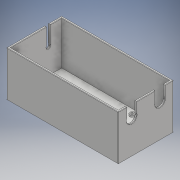
# Autodesk Inventor part: END NODE SIMPLE
Saved by Autodesk Inventor 2017 (Build 210142000, 142)
## iProperties
Created: 2019-07-16
Part Number: END NODE SIMPLE
Material: Generic
Document SubType Name: Modeling
Designer: harneet
Density: 1 g/cm^3
Appearance: Default
Author: harneet
Autodesk Inventor part; units mm, degrees
ref_plane "YZ Plane" through (0, 0, 0) normal (1, 0, 0) x (0, 1, 0)
ref_plane "XZ Plane" through (0, 0, 0) normal (0, 1, 0) x (-1, 0, 0)
ref_plane "XY Plane" through (0, 0, 0) normal (0, 0, 1) x (1, 0, 0)
sketch "Sketch1" plane through (0, 0, 0) normal (0, 0, 1) x (1, 0, 0)
  line L0 (-68.5, 32.5) -> (68.5, 32.5)
  line L1 (68.5, 32.5) -> (68.5, -32.5)
  line L2 (68.5, -32.5) -> (-68.5, -32.5)
  line L3 (-68.5, -32.5) -> (-68.5, 32.5)
  line L4 (71, 35) -> (-71, 35)
  line L5 (-71, 35) -> (-71, -35)
  line L6 (-71, -35) -> (71, -35)
  line L7 (71, -35) -> (71, 35)
  point P0 (0, 0)
  dimension "d0" = 137
  dimension "d1" = 68.5
  dimension "d2" = 65
  dimension "d3" = 32.5
  dimension "d4" = 2.5
  constraints: 16 end point, 4 parallel, 2 perpendicular, 1 horizontal, 3 other
  measures "d0" distance of L0.start L0.end
  measures "d1" distance from line of point (0, 0) L3
  measures "d2" distance of L2.end L0.start
  measures "d3" distance from line of L2 point (0, 0)
  measures "d4" distance between parallel lines of L0 L4
extrude "Extrusion1" add sketch "Sketch1" along normal blind 55
sketch "Sketch2" plane through (0, 0, 0) normal (0, 0, -1) x (-1, 0, 0)
  line L0 (71, 35) -> (-71, 35)
  line L1 (-71, 35) -> (-71, -35)
  line L2 (-71, -35) -> (71, -35)
  line L3 (71, -35) -> (71, 35)
  point P0 (0, 0)
  dimension "d7" = 142
  dimension "d8" = 70
  dimension "d9" = 35
  dimension "d10" = 71
  constraints: 8 end point, 2 parallel, 1 horizontal, 1 perpendicular
  measures "d7" distance of L1.end L2.end
  measures "d8" distance of L0.end L1.end
  measures "d9" distance from line of point (0, 0) L2
  measures "d10" distance from line of point (0, 0) L1
extrude "Extrusion2" add sketch "Sketch2" along normal blind 2.5
sketch "Sketch3" plane through (71, -35, 55) normal (1, 0, 0) x (0, 0, -1)
  circle A0 centre (15, 17) radius 6.375
  circle A1 centre (15, 53) radius 6.375
  line L0 (55, 2.5) -> (55, 67.5) projected
  line L1 (57.5, 0) -> (0, 0) projected
  point P0 (55, 35)
  dimension "d13" = 12.75
  dimension "d14" = 12.75
  dimension "d15" = 40
  dimension "d16" = 40
  dimension "d17" = 36
  dimension "d18" = 17
  constraints: 2 centre point
  measures "d13" diameter of A0
  measures "d14" diameter of A1
  measures "d15" distance from line of L0 A0.centre
  measures "d16" distance from line of A1.centre L0
  measures "d17" distance of A1.centre A0.centre
  measures "d18" distance from line of L1 A0.centre
extrude "Extrusion3" cut sketch "Sketch3" against normal up to surface (2.5 mm away)
sketch "Sketch4" plane through (-68.5, -32.5, 55) normal (1, 0, 0) x (0, 0, -1)
  circle A0 centre (23, 48) radius 2.5
  circle A1 centre (15, 50.5) radius 6.375 projected
  point P0 (55, 32.5)
  point P1 (0, 65)
  dimension "d21" = 5
  dimension "d22" = 17
  dimension "d25" = 8
  constraints: 1 centre point
  measures "d21" diameter of A0
  measures "d22" vertical distance of point (0, 65) A0.centre
  measures "d25" horizontal distance of A0.centre A1.centre
extrude "Extrusion4" cut sketch "Sketch4" against normal blind 2.5 contours A0 A1 | A1 A0 picked at (22.5229, 48.2025) picked at (20.8961, 48.5627)
sketch "Sketch5" plane through (0, 0, 0) normal (0, 0, 1) x (1, 0, 0)
  circle A0 centre (28.5, -7) radius 1.5
  circle A1 centre (28.5, -22.5) radius 1.5
  line L0 (68.5, 32.5) -> (68.5, -32.5) projected
  line L1 (68.5, -32.5) -> (-68.5, -32.5) projected
  point P0 (0, 0)
  dimension "d28" = 3
  dimension "d29" = 3
  dimension "d32" = 15.5
  dimension "d33" = 40
  dimension "d34" = 40
  dimension "d35" = 10
  constraints: 2 centre point
  measures "d28" diameter of A0
  measures "d29" diameter of A1
  measures "d32" distance of A0.centre A1.centre
  measures "d33" distance from line of A1.centre L0
  measures "d34" distance from line of L0 A0.centre
  measures "d35" distance from line of A1.centre L1
extrude "Extrusion5" cut sketch "Sketch5" against normal through all
sketch "Sketch6" plane through (0, 0, 0) normal (0, 0, 1) x (1, 0, 0)
  circle A0 centre (28.5, -7) radius 1.5 projected
  circle A1 centre (28.5, -22.5) radius 1.5 projected
  circle A2 centre (28.5, -7) radius 3
  circle A3 centre (28.5, -22.5) radius 3
  point P0 (0, 0)
  dimension "d38" = 6
  dimension "d39" = 6
  constraints: 2 centre point, 2 coincident
  measures "d38" diameter of A2
  measures "d39" diameter of A3
extrude "Extrusion6" add sketch "Sketch6" along normal blind 2.5
sketch "Sketch7" plane through (0, 0, 0) normal (0, 0, 1) x (1, 0, 0)
  circle A0 centre (28.5, 25) radius 1.5
  circle A1 centre (58.5, 25) radius 1.5
  circle A2 centre (58.5, 5) radius 1.5
  circle A3 centre (28.5, 5) radius 1.5
  line L0 (-68.5, 32.5) -> (68.5, 32.5) projected
  line L1 (68.5, 32.5) -> (68.5, -32.5) projected
  point P0 (0, 0)
  dimension "d42" = 3
  dimension "d43" = 3
  dimension "d44" = 3
  dimension "d45" = 3
  dimension "d46" = 30
  dimension "d47" = 20
  dimension "d48" = 0
  dimension "d49" = 20
  dimension "d50" = 7.5
  dimension "d51" = 10
  dimension "d52" = 0
  dimension "d53" = 0
  constraints: 4 centre point
  measures "d42" diameter of A0
  measures "d43" diameter of A1
  measures "d44" diameter of A2
  measures "d45" diameter of A3
  measures "d46" distance of A1.centre A0.centre
  measures "d47" distance of A2.centre A1.centre
  measures "d48" horizontal distance of A2.centre A1.centre
  measures "d49" distance of A3.centre A0.centre
  measures "d50" distance from line of A1.centre L0
  measures "d51" distance from line of L1 A1.centre
  measures "d52" vertical distance of A1.centre A0.centre
  measures "d53" vertical distance of A2.centre A3.centre
extrude "Extrusion7" cut sketch "Sketch7" against normal through all
sketch "Sketch8" plane through (0, 0, 0) normal (0, 0, 1) x (1, 0, 0)
  circle A0 centre (28.5, 25) radius 1.5 projected
  circle A1 centre (28.5, 5) radius 1.5 projected
  circle A2 centre (58.5, 5) radius 1.5 projected
  circle A3 centre (58.5, 25) radius 1.5 projected
  circle A4 centre (28.5, 25) radius 3
  circle A5 centre (58.5, 25) radius 3
  circle A6 centre (58.5, 5) radius 3
  circle A7 centre (28.5, 5) radius 3
  point P0 (0, 0)
  dimension "d56" = 6
  dimension "d57" = 6
  dimension "d58" = 6
  dimension "d59" = 6
  constraints: 4 centre point, 4 coincident
  measures "d56" diameter of A4
  measures "d57" diameter of A5
  measures "d58" diameter of A6
  measures "d59" diameter of A7
extrude "Extrusion8" add sketch "Sketch8" along normal blind 2.5
fillet "Fillet1" radius 0.5 28 edges at (71, 18, 46.375) (71, -18, 46.375) (68.5, -18, 46.375) (68.5, 18, 46.375) (68.5, 0, 55) (0, -32.5, 55) (-68.5, 0, 55) (0, 32.5, 55) (71, 35, 26.25) (71, 0, 55) (71, -35, 26.25) (71, 0, -2.5) (0, 35, 55) (-71, 0, 55) (0, -35, 55) (0, 35, -2.5) (0, -35, -2.5) (-71, 0, -2.5) (-71, -35, 26.25) (-71, 35, 26.25) (-71, 15.5, 34.5) (-68.5, 15.5, 34.5) (57, 5, -2.5) (57, 25, -2.5) (27, 25, -2.5) (27, 5, -2.5) (27, -7, -2.5) (27, -22.5, -2.5)
fillet "Fillet2" radius 0.5 6 edges at (25.5, -22.5, 2.5) (25.5, -7, 2.5) (25.5, 5, 2.5) (25.5, 25, 2.5) (55.5, 5, 2.5) (55.5, 25, 2.5)
sketch "Sketch9" plane through (71, -34.5, 54.5) normal (1, 0, 0) x (0, 0, -1)
  circle A0 centre (14.5, 16.5) radius 6.875 projected
  circle A1 centre (14.5, 52.5) radius 6.875 projected
  line L0 (0, 69) -> (56.5, 69) projected
  line L1 (0, 0) -> (0, 69) projected
  line L2 (56.5, 0) -> (0, 0) projected
  line L3 (56.5, 69) -> (56.5, 0) projected
  line L4 (-0.5, 10.125) -> (14.5, 10.125)
  line L5 (-0.5, 69) -> (-0.5, 0) projected
  circle A2 centre (14.5, 16.5) radius 6.375 projected
  circle A3 centre (14.5, 52.5) radius 6.375 projected
  arc A4 (14.5, 22.875) -> (14.5, 10.125) centre (14.5, 16.5) ccw
  arc A5 (14.5, 58.875) -> (14.5, 46.125) centre (14.5, 52.5) ccw
  line L6 (-0.5, 22.875) -> (14.5, 22.875)
  line L7 (-0.5, 46.125) -> (14.5, 46.125)
  line L8 (-0.5, 58.875) -> (14.5, 58.875)
  line L9 (-0.5, 46.125) -> (-0.5, 58.875)
  line L10 (-0.5, 10.125) -> (-0.5, 22.875)
  point P0 (54.5, 34.5)
  constraints: 12 end point, 4 point on circle, 4 point on line, 4 tangent, 3 horizontal, 2 centre point, 2 coincident, 2 collinear, 2 concentric, 1 perpendicular
extrude "Extrusion10" cut sketch "Sketch9" against normal blind 2.5 contours L6 A2 L4 A0 | A0 L4 L1 L6 | L1 L4 L5 L6 | L7 L5 L8 L1 | L1 L8 A1 L7 | A1 L8 A3 L7 picked at (7.9893, 16.5) picked at (7.9893, 52.5)
sketch "Sketch10" plane through (-71, -34.5, -2) normal (-1, 0, 0) x (0, 0, 1)
  line L0 (57, 0) -> (57, 69) projected
  line L1 (56.5, 69.5) -> (0, 69.5) projected
  circle A0 centre (34, 50) radius 2.5 projected
  arc A1 (34, 47.5) -> (34, 52.5) centre (34, 50) ccw
  line L2 (57, 52.5) -> (34, 52.5)
  line L3 (57, 47.5) -> (34, 47.5)
  point P0 (2, 34.5)
  dimension "d72" = 17
  constraints: 4 end point, 2 point on circle, 2 point on line, 1 centre point, 1 coincident, 1 concentric, 1 horizontal, 1 perpendicular, 1 tangent
  measures "d72" distance between parallel lines of L1 L2
extrude "Extrusion11" cut sketch "Sketch10" against normal blind 2.5 contours L3 A0 L2 L0
equation "\"d1\" = 0.5 * d0"
equation "\"d3\" = 0.5 * d2"
equation "\"d14\" = d13"
equation "\"d16\" = d15"
equation "\"d34\" = d33"
equation "\"d49\" = d47"
body "Solid1"
